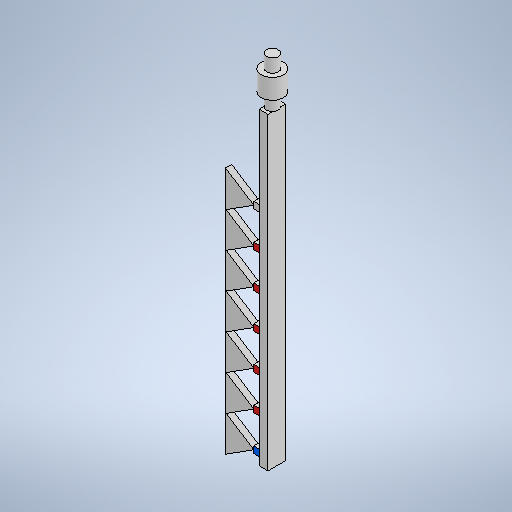
# Autodesk Inventor part: ДМФ 081 труба форсунки v2.0
Saved by Autodesk Inventor 2026.2 (Build 302298010, 298A)
## iProperties
Created: 2024-06-28
Part Number: ДМФ 081 труба форсунки v2.0
Material: Generic
Document SubType Name: Modeling
Designer: admin
Density: 1 g/cm^3
Appearance: Default
Author: admin
Autodesk Inventor part; units mm, degrees
ref_plane "YZ Plane" through (0, 0, 0) normal (1, 0, 0) x (0, 1, 0)
ref_plane "XZ Plane" through (0, 0, 0) normal (0, 1, 0) x (-1, 0, 0)
ref_plane "XY Plane" through (0, 0, 0) normal (0, 0, 1) x (1, 0, 0)
sketch "Sketch2" plane through (0, 0, 0) normal (0, 0, 1) x (1, 0, 0)
  line L0 (-10, 20) -> (10, 20)
  line L1 (10, 20) -> (10, -20)
  line L2 (10, -20) -> (-10, -20)
  line L3 (-10, -20) -> (-10, 20)
  line L4 (-10, 20) -> (10, -20) construction
  line L5 (10, 20) -> (-10, -20) construction
  point P0 (0, 0)
  dimension "d8" = 20
  dimension "d9" = 40
  constraints: 12 end point, 2 midpoint, 2 parallel, 1 horizontal, 1 perpendicular
  measures "d8" distance of L1.end L2.end
  measures "d9" distance of L0.end L1.end
extrude "Extrusion2" add sketch "Sketch2" against normal blind 700
sketch "Sketch3" plane through (0, 0, 0) normal (0, 1, 0) x (-1, 0, 0)
  line L0 (10, 0) -> (-10, 0) construction
  line L1 (10, 0) -> (10, -700) construction
  line L2 (-10, -700) -> (10, -700) construction
  line L3 (-10, 0) -> (-10, -700) construction
  line L4 (10, -680) -> (35, -680)
  line L5 (35, -680) -> (35, -695)
  line L6 (35, -695) -> (10, -695)
  line L7 (10, -695) -> (10, -680)
  line L8 (35, -687.5) -> (99.3571, -687.5)
  line L9 (35, -687.5) -> (99.3571, -646.5)
  line L10 (35, -687.5) -> (99.3571, -728.5)
  line L11 (99.3571, -728.5) -> (99.3571, -646.5)
  point P0 (0, 0)
  dimension "d21" = 25
  dimension "d22" = 15
  dimension "d23" = 5
  dimension "d24" = 65
  dimension "d25" = 82
  dimension "d26" = 64.3571
  dimension "d27" = 109.3571
  constraints: 18 end point, 2 horizontal, 2 midpoint, 2 parallel, 1 perpendicular, 1 point on line, 1 vertical
  measures "d21" distance of L5.end L6.end
  measures "d22" distance between parallel lines of L6 L4
  measures "d23" distance between parallel lines of L2 L6
  measures "d24" angle of L10 L9
  measures "d25" distance of L10.end L9.end
  measures "d26" distance between parallel lines of L5 L11
  measures "d27" distance between parallel lines of L11 L3
extrude "Extrusion3" add sketch "Sketch3" along normal mid plane 14
pattern_linear "Rectangular Pattern1" count 7 spacing 80 along (0, 0, 1) of "Extrusion3"
sketch "Sketch4" plane through (0, 0, 0) normal (1, 0, 0) x (0, 1, 0)
  line L0 (0, 0) -> (0, 105)
  line L1 (0, 105) -> (-13.5, 105)
  line L2 (-13.5, 105) -> (-13.5, 75)
  line L3 (-13.5, 75) -> (-25, 75)
  line L4 (-25, 75) -> (-25, 30)
  line L5 (-25, 30) -> (-13.5, 30)
  line L6 (-13.5, 30) -> (-13.5, 0)
  line L7 (-7, -200) -> (-7, -215) projected
  line L8 (-7, -215) -> (7, -215) projected
  line L9 (7, -215) -> (7, -200) projected
  line L10 (7, -200) -> (-7, -200) projected
  line L11 (-7, -280) -> (-7, -295) projected
  line L12 (-7, -295) -> (7, -295) projected
  line L13 (7, -295) -> (7, -280) projected
  line L14 (7, -280) -> (-7, -280) projected
  line L15 (-7, -360) -> (-7, -375) projected
  line L16 (-7, -375) -> (7, -375) projected
  line L17 (7, -375) -> (7, -360) projected
  line L18 (7, -360) -> (-7, -360) projected
  line L19 (-7, -440) -> (-7, -455) projected
  line L20 (-7, -455) -> (7, -455) projected
  line L21 (7, -455) -> (7, -440) projected
  line L22 (7, -440) -> (-7, -440) projected
  line L23 (-7, -520) -> (-7, -535) projected
  line L24 (-7, -535) -> (7, -535) projected
  line L25 (7, -535) -> (7, -520) projected
  line L26 (7, -520) -> (-7, -520) projected
  line L27 (-7, -600) -> (-7, -615) projected
  line L28 (-7, -615) -> (7, -615) projected
  line L29 (7, -615) -> (7, -600) projected
  line L30 (7, -600) -> (-7, -600) projected
  line L31 (-7, -680) -> (-7, -695) projected
  line L32 (-7, -695) -> (7, -695) projected
  line L33 (7, -695) -> (7, -680) projected
  line L34 (7, -680) -> (-7, -680) projected
  line L35 (20, 0) -> (-20, 0) projected
  line L36 (20, 0) -> (20, -700) projected
  line L37 (-20, -700) -> (20, -700) projected
  line L38 (-20, 0) -> (-20, -700) projected
  dimension "d28" = 105
  dimension "d29" = 30
  dimension "d30" = 30
  dimension "d31" = 50
  dimension "d32" = 27
  constraints: 14 end point, 6 perpendicular, 2 point on line, 2 vertical
  measures "d28" distance of L0.start L0.end
  measures "d29" distance of L1.end L2.end
  measures "d30" distance of L6.end L5.end
  measures "d31" diameter of L4 L0
  measures "d32" diameter of L2 L0
revolve "Revolution1" add sketch "Sketch4" angle 360 about axis through (0, 0, 0) along (0, 0, 1) contours L35 L6 L5 L4 L3 L2 L1 L0
equation "\"d30\" = d29"
body "Solid2"
